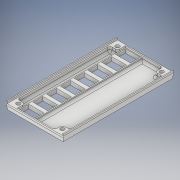
# Autodesk Inventor part: LineSensorGuard_sa
Saved by Autodesk Inventor 2019 (Build 230136000, 136)
## iProperties
Created: 2019-01-11
Part Number: LineSensorGuard_sa
Material: ABS プラスチック
Document SubType Name: Modeling
Designer: shun
Density: 1.06 g/cm^3
Appearance: 滑らか - 白
Author: shun
Autodesk Inventor part; units mm, degrees
ref_plane "YZ Plane" through (0, 0, 0) normal (1, 0, 0) x (0, 1, 0)
ref_plane "XZ Plane" through (0, 0, 0) normal (0, 1, 0) x (-1, 0, 0)
ref_plane "XY Plane" through (0, 0, 0) normal (0, 0, 1) x (1, 0, 0)
sketch "スケッチ1" plane through (0, 0, 0) normal (0, 1, 0) x (-1, 0, 0)
  line L0 (25, 50) -> (-25, 50)
  line L1 (-25, 50) -> (-25, -50)
  line L2 (-25, -50) -> (25, -50)
  line L3 (25, -50) -> (25, 50)
  line L4 (25, 50) -> (-25, -50) construction
  line L5 (-25, 50) -> (25, -50) construction
  line L6 (25, 50) -> (17, 50)
  line L7 (17, 50) -> (17, 44)
  line L8 (19, 42) -> (25, 42)
  line L9 (25, 42) -> (25, 50)
  line L10 (20, 45) -> (-20, 45) construction
  line L11 (-20, 45) -> (-20, -45) construction
  line L12 (-20, -45) -> (20, -45) construction
  line L13 (20, -45) -> (20, 45) construction
  line L14 (25, -50) -> (17, -50)
  line L15 (17, -50) -> (17, -44)
  line L16 (19, -42) -> (25, -42)
  line L17 (25, -42) -> (25, -50)
  line L18 (-25, -50) -> (-17, -50)
  line L19 (-17, -50) -> (-17, -44)
  line L20 (-19, -42) -> (-25, -42)
  line L21 (-25, -42) -> (-25, -50)
  line L22 (-25, 50) -> (-17, 50)
  line L23 (-17, 50) -> (-17, 44)
  line L24 (-19, 42) -> (-25, 42)
  line L25 (-25, 42) -> (-25, 50)
  arc A0 (-19, 42) -> (-17, 44) centre (-19, 44) ccw
  arc A1 (-17, -44) -> (-19, -42) centre (-19, -44) ccw
  arc A2 (19, -42) -> (17, -44) centre (19, -44) ccw
  arc A3 (17, 44) -> (19, 42) centre (19, 44) ccw
  point P0 (0, 0)
  point P1 (17, 42)
  point P2 (17, -42)
  point P3 (-17, -42)
  point P4 (-17, 42)
  dimension "d0" = 50
  dimension "d1" = 100
  dimension "d2" = 8
  dimension "d3" = 8
  dimension "d4" = 5
  dimension "d5" = 8
  dimension "d6" = 8
  dimension "d7" = 8
  dimension "d8" = 8
  dimension "d9" = 8
  dimension "d10" = 8
  dimension "d11" = 2
  constraints: 52 end point, 12 parallel, 8 point on circle, 8 point on line, 8 tangent, 6 perpendicular, 5 horizontal, 4 centre point, 4 coincident, 3 equal radius, 2 midpoint, 3 other
  measures "d0" distance of L2.end L1.end
  measures "d1" distance of L1.end L0.end
  measures "d2" distance of L8.end point (17, 42)
  measures "d3" distance of point (17, 42) L6.end
  measures "d4" distance between parallel lines of L3 L13
  measures "d5" distance of point (17, -42) L16.end
  measures "d6" distance of L14.end point (17, -42)
  measures "d7" distance of L20.end point (-17, -42)
  measures "d8" distance of point (-17, -42) L18.end
  measures "d9" distance of point (-17, 42) L24.end
  measures "d10" distance of L22.end point (-17, 42)
  measures "d11" radius of A0
extrude "押し出し1" add sketch "スケッチ1" along normal blind 4.5 contours L3 L8 A3 L7 L0 | L23 A0 L24 L1 L0 | L3 L2 L15 A2 L16 | L20 A1 L19 L2 L1
sketch "スケッチ2" plane through (17, 0, 50) normal (0, 0, 1) x (1, 0, 0)
  line L0 (-42, 0) -> (-42, 4.5) projected
  line L1 (-17, 0) -> (-42, 0)
  line L2 (-17, 0) -> (-17, -0.6)
  line L3 (-17, -0.6) -> (-42, -0.6)
  line L4 (-42, -0.6) -> (-42.1, -0.6)
  line L5 (-42, 4.5) -> (-43, 4.5)
  line L6 (-43, 4.5) -> (-42.1, -0.6)
  dimension "d16" = 0.6
  dimension "d17" = 0.1
  dimension "d18" = 1
  constraints: 12 end point, 2 perpendicular, 2 point on line, 1 horizontal, 1 vertical
  measures "d16" distance of L1.start L2.end
  measures "d17" distance of L3.end L4.end
  measures "d18" distance of L0.end L5.end
extrude "押し出し2" add sketch "スケッチ2" against normal blind 100
mirror "ミラー1" about plane through (0, 0, 50) normal (1, 0, 0) of "押し出し2"
sketch "スケッチ3" plane through (-17, 0, 50) normal (0, 1, 0) x (1, 0, 0)
  line L0 (0, 0) -> (0, 6) projected
  line L1 (34, 6) -> (34, 0) projected
  line L2 (0, 0) -> (34, 0)
  line L3 (34, 0) -> (34, 1)
  line L4 (34, 1) -> (0, 1)
  line L5 (0, 1) -> (0, 0)
  point P0 (17, 50)
  dimension "d21" = 1
  constraints: 8 end point, 2 parallel, 1 horizontal, 1 perpendicular, 1 point on line
  measures "d21" distance of L3.end L2.end
extrude "押し出し3" add sketch "スケッチ3" along normal up to surface (4.5 mm away)
mirror "ミラー2" about plane through (0, 0, 0) normal (0, 0, 1) of "押し出し3"
sketch "スケッチ4" plane through (-25, 0, -42) normal (0, 1, 0) x (1, 0, 0)
  line L0 (8.9, -2.75) -> (22.4, -2.75)
  line L1 (22.4, -2.75) -> (22.4, 6.25)
  line L2 (22.4, 6.25) -> (8.9, 6.25)
  line L3 (8.9, 6.25) -> (8.9, -2.75)
  line L4 (8.9, -2.75) -> (22.4, 6.25) construction
  line L5 (22.4, -2.75) -> (8.9, 6.25) construction
  line L6 (51, 8) -> (-1, 8) projected
  line L7 (-0.1, -92) -> (-0.1, 8) projected
  point P0 (25, -42)
  point P1 (15.65, 1.75)
  dimension "d24" = 13.5
  dimension "d25" = 9
  dimension "d26" = 6.25
  dimension "d27" = 9
  constraints: 12 end point, 2 midpoint, 2 parallel, 1 horizontal, 1 perpendicular
  measures "d24" distance of L2.end L1.end
  measures "d25" distance of L1.end L0.end
  measures "d26" distance from line of L6 point (15.65, 1.75)
  measures "d27" distance between parallel lines of L7 L3
extrude "押し出し4" cut sketch "スケッチ4" against normal blind 1
pattern_linear "矩形状パターン1" count 8 spacing 12.5 along (0, 0, 1) of "押し出し4"
hole "穴1" at (-20, 0, 45) at (-20, 0, -45) at (20, 0, -45) at (20, 0, 45) direction (0, -1, 0) diameter 3.6 end through all both
sketch "スケッチ6" plane through (-25, 0, -42) normal (0, 0, 1) x (1, 0, 0)
  line L0 (0, 4.5) -> (6, 4.5) projected
  line L1 (0, 0) -> (6, 0) projected
  line L2 (0, 4.5) -> (1, 4.5)
  line L3 (1, 4.5) -> (1, 0)
  line L4 (1, 0) -> (0, 0)
  line L5 (0, 0) -> (0, 4.5)
  line L6 (44, 4.5) -> (50, 4.5) projected
  line L7 (50, 4.5) -> (49, 4.5)
  line L8 (49, 4.5) -> (49, 0)
  line L9 (49, 0) -> (50, 0)
  line L10 (50, 0) -> (50, 4.5)
  point P0 (25, 0)
  dimension "d57" = 1
  dimension "d58" = 1
  constraints: 16 end point, 4 parallel, 2 horizontal, 2 perpendicular, 2 point on line
  measures "d57" distance of L3.end L4.end
  measures "d58" distance of L9.end L8.end
extrude "押し出し6" add sketch "スケッチ6" along normal up to surface (84 mm away)
sketch "スケッチ7" plane through (-17, 0, 49) normal (0, 1, 0) x (1, 0, 0)
  line L0 (14.4, 97.25) -> (14.4, 88.25) projected
  line L1 (14.4, 88.25) -> (0.9, 88.25) projected
  line L2 (0.9, 88.25) -> (0.9, 97.25) projected
  line L3 (0.9, 97.25) -> (14.4, 97.25) projected
  line L4 (0, 93) -> (0, 98) projected
  line L5 (0, 0) -> (34, 0) projected
  line L6 (0, 98) -> (15.4, 98)
  line L7 (15.4, 98) -> (15.4, 0)
  line L8 (15.4, 0) -> (0, 0)
  line L9 (0, 0) -> (0, 98)
  line L10 (-7, 91) -> (-7, 7) projected
  line L11 (-2, 7) -> (-7, 7) projected
  arc A0 (0, 5) -> (-2, 7) centre (-2, 5) ccw projected
  line L12 (0, 0) -> (0, 5) projected
  line L13 (0, 0) -> (34, 0) projected
  line L14 (34, 5) -> (34, 0) projected
  arc A1 (36, 7) -> (34, 5) centre (36, 5) ccw projected
  line L15 (41, 7) -> (36, 7) projected
  line L16 (41, 7) -> (41, 91) projected
  line L17 (36, 91) -> (41, 91) projected
  arc A2 (34, 93) -> (36, 91) centre (36, 93) ccw projected
  line L18 (34, 98) -> (34, 93) projected
  line L19 (34, 98) -> (0, 98) projected
  line L20 (0, 93) -> (0, 98) projected
  arc A3 (-2, 91) -> (0, 93) centre (-2, 93) ccw projected
  line L21 (-7, 91) -> (-2, 91) projected
  line L22 (14.4, 9.75) -> (14.4, 0.75) projected
  line L23 (14.4, 0.75) -> (0.9, 0.75) projected
  line L24 (0.9, 0.75) -> (0.9, 9.75) projected
  line L25 (0.9, 9.75) -> (14.4, 9.75) projected
  line L26 (14.4, 22.25) -> (14.4, 13.25) projected
  line L27 (14.4, 13.25) -> (0.9, 13.25) projected
  line L28 (0.9, 13.25) -> (0.9, 22.25) projected
  line L29 (0.9, 22.25) -> (14.4, 22.25) projected
  line L30 (14.4, 34.75) -> (14.4, 25.75) projected
  line L31 (14.4, 25.75) -> (0.9, 25.75) projected
  line L32 (0.9, 25.75) -> (0.9, 34.75) projected
  line L33 (0.9, 34.75) -> (14.4, 34.75) projected
  line L34 (14.4, 47.25) -> (14.4, 38.25) projected
  line L35 (14.4, 38.25) -> (0.9, 38.25) projected
  line L36 (0.9, 38.25) -> (0.9, 47.25) projected
  line L37 (0.9, 47.25) -> (14.4, 47.25) projected
  line L38 (14.4, 59.75) -> (14.4, 50.75) projected
  line L39 (14.4, 50.75) -> (0.9, 50.75) projected
  line L40 (0.9, 50.75) -> (0.9, 59.75) projected
  line L41 (0.9, 59.75) -> (14.4, 59.75) projected
  line L42 (14.4, 72.25) -> (14.4, 63.25) projected
  line L43 (14.4, 63.25) -> (0.9, 63.25) projected
  line L44 (0.9, 63.25) -> (0.9, 72.25) projected
  line L45 (0.9, 72.25) -> (14.4, 72.25) projected
  line L46 (14.4, 84.75) -> (14.4, 75.75) projected
  line L47 (14.4, 75.75) -> (0.9, 75.75) projected
  line L48 (0.9, 75.75) -> (0.9, 84.75) projected
  line L49 (0.9, 84.75) -> (14.4, 84.75) projected
  line L50 (14.4, 97.25) -> (14.4, 88.25) projected
  line L51 (14.4, 88.25) -> (0.9, 88.25) projected
  line L52 (0.9, 88.25) -> (0.9, 97.25) projected
  line L53 (0.9, 97.25) -> (14.4, 97.25) projected
  line L54 (14.4, 63.25) -> (14.4, 72.25) projected
  point P0 (17, 49)
  dimension "d61" = 1
  constraints: 8 end point, 2 parallel, 1 horizontal, 1 perpendicular, 1 point on line
  measures "d61" distance between parallel lines of L7 L54
extrude "押し出し7" add sketch "スケッチ7" along normal blind 3 contours L4 L6 L7 L5 L9
sketch "スケッチ8" plane through (0, 4.5, 0) normal (0, 1, 0) x (1, 0, 0)
  line L0 (-26, -50) -> (-26, 50) projected
  line L1 (-25.1, 50) -> (25.1, 50) projected
  line L2 (-26, -50) -> (-25.1, -50)
  line L3 (-25.1, -50) -> (-25.1, 50)
  line L4 (-25.1, 50) -> (-26, 50)
  line L5 (-26, 50) -> (-26, -50)
  line L6 (26, -50) -> (26, 50) projected
  line L7 (25.1, -50) -> (25.1, 50) projected
  line L8 (26, -50) -> (25.1, -50)
  line L9 (25.1, -50) -> (25.1, 50)
  line L10 (25.1, 50) -> (26, 50)
  line L11 (26, 50) -> (26, -50)
  point P0 (0, 0)
  dimension "d64" = 0.9
  dimension "d65" = 0.9
  constraints: 16 end point, 4 parallel, 2 horizontal, 2 perpendicular
  measures "d64" distance of L4.end L1.start
  measures "d65" distance of L1.end L10.end
extrude "押し出し8" add sketch "スケッチ8" along normal blind 1.5
fillet "フィレット2" radius 2 21 edges at (-17.5858, 0, 42.5858) (-21.5, 0, 42) (-24, 0, 0) (-17.5858, 0, -42.5858) (-21.5, 0, -42) (-24, 2.25, -42) (-24, 2.25, 42) (24, 0, 0) (24, 2.25, -42) (24, 2.25, 42) (17, 2.25, 49) (17.5858, 0, 42.5858) (21.5, 0, 42) (17, 0, 46.5) (7.7, 0, 49) (17, 2.25, -49) (7.7, 0, -49) (17.5858, 0, -42.5858) (21.5, 0, -42) (17, 0, -46.5) (-1.6, 0, 0)
chamfer "面取り2" distance 0.5 distance2 3.4 1 edges at (0, -0.6, -50) measured on face at (0, -0.6, -49.5)
chamfer "面取り3" distance 3.4 distance2 0.5 1 edges at (0, -0.6, 50) measured on face at (0, -0.1, 50)
chamfer "面取り4" distance 2 angle 45 4 edges at (20, -0.6, 43.2) (20, -0.6, -46.8) (-20, -0.6, -46.8) (-20, -0.6, 43.2)
equation "\"d58\" = d57"
